Autodesk Fusion 360 part; units mm, degrees
note: some values were not read from the file. Set by a fixed rule: which sketch regions a step uses.
(part 2 of 2)
  circle A929 centre (73.5725, -9.1918) radius 2.5
  circle A930 centre (73.6938, -15.3062) radius 2.5
  circle A931 centre (80.5725, -9.1918) radius 2.5
  point P0 (-62.9957, -145.0372)
  point P1 (82.0043, -145.0372)
  point P2 (-62.9957, -0.0372)
  dimension "d18" = 145
  dimension "d19" = 145
  dimension "d20" = 5
  dimension "d22" = 10
  dimension "d23" = 10
  dimension "d24" = 10
  dimension "d25" = 10
  dimension "d26" = 5
  dimension "d29" = 5
  dimension "d30" = 5
  dimension "d33" = 7
  dimension "d34" = 6
  constraint horizontal L0
  constraint vertical L1
  constraint horizontal L2
  constraint vertical L3
  constraint coincident P0 L0
  constraint coincident P0 L3
  constraint tangent L0 A0
  constraint tangent L3 A0
  constraint coincident P1 L0
  constraint coincident P1 L1
  constraint tangent L0 A1
  constraint tangent L1 A1
  constraint equal A0 A1
  constraint tangent L1 A2
  constraint tangent L2 A2
  constraint equal A0 A2
  constraint coincident P2 L2
  constraint coincident P2 L3
  constraint tangent L2 A3
  constraint tangent L3 A3
  constraint equal A0 A3
  constraint tangent L4 A4
  constraint tangent L7 A4
  constraint tangent L4 A5
  constraint tangent L5 A5
  constraint equal A4 A5
  constraint tangent L5 A6
  constraint tangent L6 A6
  constraint equal A4 A6
  constraint tangent L6 A7
  constraint tangent L7 A7
  constraint equal A4 A7
  measures "d18" distance of P0 P1
  measures "d19" distance of P0 P2
  measures "d20" radius of A0
  measures "d22" distance of L0 L4
  measures "d23" distance of L1 L5
  measures "d24" distance of L2 L6
  measures "d25" distance of L3 L7
  measures "d26" radius of A4
  measures "d29" diameter of A8
  measures "d30" diameter of A9
extrude "Extrude2" add sketch "Sketch2" along normal blind 100 contours L0 L1 L2 L3 A0 A1 A2 A3 A51 A93 A135 A177 A219 A261 A303 A345 A387 A429 A469 A511 A553 A595 A637 A679 A721 A763 A805 A847 A889 A931 | L1 A51 | L1 A93 | L1 A931 | L1 A135 | L1 A889 | L1 A177 | L1 A847 | L1 A219 | L1 A805 | L1 A261 | L1 A763 | L1 A303 | L1 A721 | L1 A345 | L1 A679 | L1 A387 | L1 A637 | L1 A429 | L1 A595 | L1 A469 | L1 A553 | L1 A511 | L4 A15 A58 | A4 A13 A56 | L4 A15 A58 | L4 A15 A58 | A4 A13 A56 | A4 A13 A56 | L4 A17 A60 | A4 A55 A98 | L4 A17 A60 | L4 A17 A60 | L7 A4 A55 A98 | L7 A55 A98 | L4 A19 A62 | L7 A97 A140 | L4 A19 A62 | L4 A19 A62 | L7 A97 A140 | L7 A97 A140 | L4 A21 A64 | L7 A139 A182 | L4 A21 A64 | L4 A21 A64 | L7 A139 A182 | L7 A139 A182 | L4 A23 A66 | L7 A181 A224 | L4 A23 A66 | L4 A23 A66 | L7 A181 A224 | L7 A181 A224 | L4 A25 A68 | L7 A223 A266 | L4 A25 A68 | L4 A25 A68 | L7 A223 A266 | L7 A223 A266 | L4 A27 A70 | L7 A265 A308 | L4 A27 A70 | L4 A27 A70 | L7 A265 A308 | L7 A265 A308 | L4 A29 A72 | L7 A307 A350 | L4 A29 A72 | L4 A29 A72 | L7 A307 A350 | L7 A307 A350 | L4 A31 A74 | L7 A349 A392 | L4 A31 A74 | L4 A31 A74 | L7 A349 A392 | L7 A349 A392 | L4 A33 A76 | L7 A391 A434 | L4 A33 A76 | L4 A33 A76 | L7 A391 A434 | L7 A391 A434 | L4 A35 A78 | L7 A433 A474 | L4 A35 A78 | L4 A35 A78 | L7 A433 A474 | L7 A433 A474 | L4 A37 A80 | L7 A473 A516 | L4 A37 A80 | L4 A37 A80 | L7 A473 A516 | L7 A473 A516 | L4 A39 A82 | L7 A515 A558 | L4 A39 A82 | L4 A39 A82 | L7 A515 A558 | L7 A515 A558 | L4 A41 A84 | L7 A557 A600 | L4 A41 A84 | L4 A41 A84 | L7 A557 A600 | L7 A557 A600 | L4 A43 A86 | L7 A599 A642 | L4 A43 A86 | L4 A43 A86 | L7 A599 A642 | L7 A599 A642 | L4 A45 A88 | L7 A641 A684 | L4 A45 A88 | L4 A45 A88 | L7 A641 A684 | L7 A641 A684 | L4 A47 A90 | L7 A683 A726 | L4 A5 A47 A90 | A5 A47 A90 | L7 A683 A726 | L7 A683 A726 | L5 A5 A91 A134 | L7 A725 A768 | L5 A91 A134 | A91 A134 | L7 A725 A768 | L7 A725 A768 | L5 A133 A176 | L5 A133 A176 | L7 A767 A810 | L5 A133 A176 | L7 A767 A810 | L7 A767 A810 | L5 A175 A218 | L5 A175 A218 | L7 A809 A852 | L5 A175 A218 | L7 A809 A852 | L7 A809 A852 | L5 A217 A260 | L5 A217 A260 | L7 A851 A894 | L5 A217 A260 | L7 A7 A851 A894 | A7 A851 A894 | L5 A259 A302 | L5 A259 A302 | A7 A893 | L5 A259 A302 | L5 A301 A344 | L5 A301 A344 | L6 A895 | L5 A301 A344 | L5 A343 A386 | L6 A897 | L5 A343 A386 | L5 A343 A386 | L6 A899 | L5 A385 A428 | L5 A385 A428 | L6 A901 | L5 A385 A428 | L5 A427 A468 | L6 A903 | L5 A427 A468 | L5 A427 A468 | L6 A905 | L5 A467 A510 | L5 A467 A510 | L6 A907 | L5 A467 A510 | L5 A509 A552 | L6 A909 | L5 A509 A552 | L5 A509 A552 | L6 A911 | L5 A551 A594 | L5 A551 A594 | L6 A913 | L5 A551 A594 | L5 A593 A636 | L6 A915 | L5 A593 A636 | L5 A593 A636 | L6 A917 | L5 A635 A678 | L5 A635 A678 | L6 A919 | L5 A635 A678 | L5 A677 A720 | L6 A921 | L5 A677 A720 | L5 A677 A720 | L6 A923 | L5 A719 A762 | L5 A719 A762 | L6 A925 | L5 A719 A762 | L5 A761 A804 | L6 A6 A927 | L5 A761 A804 | L5 A761 A804 | A6 A887 A930 | L5 A803 A846 | L5 A6 A887 A930 | L5 A887 A930 | L5 A803 A846 | L5 A803 A846 | L5 A845 A888 | L5 A845 A888 | L5 A845 A888 | A11 A54 | A11 A54 | A11 A54 | A12 | A14 | A16 | A18 | A20 | A22 | A24 | A26 | A28 | A30 | A32 | A34 | A36 | A38 | A40 | A42 | A44 | A46 | A48 | A49 A92 | A49 A92 | A49 A92 | A50 | A53 A96 | A53 A96 | A53 A96 | A95 A138 | A95 A138 | A95 A138 | A137 A180 | A137 A180 | A137 A180 | A179 A222 | A179 A222 | A179 A222 | A221 A264 | A221 A264 | A221 A264 | A263 A306 | A263 A306 | A263 A306 | A305 A348 | A305 A348 | A305 A348 | A347 A390 | A347 A390 | A347 A390 | A389 A432 | A389 A432 | A389 A432 | A431 A472 | A431 A472 | A431 A472 | A471 A514 | A471 A514 | A471 A514 | A513 A556 | A513 A556 | A513 A556 | A555 A598 | A555 A598 | A555 A598 | A597 A640 | A597 A640 | A597 A640 | A639 A682 | A639 A682 | A639 A682 | A681 A724 | A681 A724 | A681 A724 | A723 A766 | A723 A766 | A723 A766 | A765 A808 | A765 A808 | A765 A808 | A807 A850 | A807 A850 | A807 A850 | A849 A892 | A849 A892 | A849 A892 | A891 | A929 picked at (80.7025, -135.0711) picked at (80.7025, -129.0711) picked at (80.7025, -9.0711) picked at (80.7025, -123.3125) picked at (80.7025, -15.3125) picked at (80.7025, -117.3125) picked at (80.7025, -21.3125) picked at (80.7025, -111.3125) picked at (80.7025, -27.3125) picked at (80.7025, -105.3125) picked at (80.7025, -33.3125) picked at (80.7025, -99.3125) picked at (80.7025, -39.3125) picked at (80.7025, -93.3125) picked at (80.7717, -45.5438) picked at (80.7025, -87.3125) picked at (80.7717, -51.5438) picked at (80.7025, -81.3125) picked at (80.7025, -57.3125) picked at (80.7025, -75.3125) picked at (80.7025, -63.3125) picked at (80.7025, -69.3125) picked at (-47.8787, -135.1454) picked at (-50.3662, -136.693) picked at (-44.5574, -135.2593) picked at (-43.3662, -136.693) picked at (-53.1044, -135.9845) picked at (-54.0864, -133.4039) picked at (-40.8787, -135.1454) picked at (-52.9107, -131.6684) picked at (-37.5574, -135.2593) picked at (-36.3662, -136.693) picked at (-53.4273, -130.4717) picked at (-54.1416, -127.5346) picked at (-33.8787, -135.1454) picked at (-53.0957, -125.6459) picked at (-30.5574, -135.2593) picked at (-29.3662, -136.693) picked at (-53.1114, -122.5202) picked at (-54.1416, -121.5346) picked at (-26.8787, -135.1454) picked at (-53.0957, -119.6459) picked at (-23.5574, -135.2593) picked at (-22.3662, -136.693) picked at (-53.1114, -116.5202) picked at (-54.1416, -115.5346) picked at (-19.8787, -135.1454) picked at (-53.0957, -113.6459) picked at (-16.5574, -135.2593) picked at (-15.3662, -136.693) picked at (-53.1114, -110.5202) picked at (-54.1416, -109.5346) picked at (-12.8787, -135.1454) picked at (-53.0957, -107.6459) picked at (-9.5574, -135.2593) picked at (-8.3662, -136.693) picked at (-53.1114, -104.5202) picked at (-54.1416, -103.5346) picked at (-5.8787, -135.1454) picked at (-53.0957, -101.6459) picked at (-2.5574, -135.2593) picked at (-1.3662, -136.693) picked at (-53.1114, -98.5202) picked at (-54.1416, -97.5346) picked at (1.1213, -135.1454) picked at (-53.0957, -95.6459) picked at (4.4426, -135.2593) picked at (5.6338, -136.693) picked at (-53.1114, -92.5202) picked at (-54.1416, -91.5346) picked at (8.1213, -135.1454) picked at (-53.0957, -89.6459) picked at (11.4426, -135.2593) picked at (12.6338, -136.693) picked at (-53.1114, -86.5202) picked at (-54.1416, -85.5346) picked at (15.1213, -135.1454) picked at (-53.0957, -83.6459) picked at (18.4426, -135.2593) picked at (19.6338, -136.693) picked at (-53.1114, -80.5202) picked at (-54.1416, -79.5346) picked at (22.1213, -135.1454) picked at (-53.0957, -77.6459) picked at (25.4426, -135.2593) picked at (26.6338, -136.693) picked at (-53.1114, -74.5202) picked at (-54.1416, -73.5346) picked at (29.1213, -135.1454) picked at (-53.0957, -71.6459) picked at (32.4426, -135.2593) picked at (33.6338, -136.693) picked at (-53.1114, -68.5202) picked at (-54.1416, -67.5346) picked at (36.1213, -135.1454) picked at (-53.0957, -65.6459) picked at (39.4426, -135.2593) picked at (40.6338, -136.693) picked at (-53.1114, -62.5202) picked at (-54.1416, -61.5346) picked at (43.1213, -135.1454) picked at (-53.0957, -59.6459) picked at (46.4426, -135.2593) picked at (47.6338, -136.693) picked at (-53.1114, -56.5202) picked at (-54.1416, -55.5346) picked at (50.1213, -135.1454) picked at (-53.0957, -53.6459) picked at (53.4426, -135.2593) picked at (54.6338, -136.693) picked at (-53.1114, -50.5202) picked at (-54.1416, -49.5346) picked at (57.1213, -135.1454) picked at (-53.0957, -47.6459) picked at (60.4426, -135.2593) picked at (61.6338, -136.693) picked at (-53.1114, -44.5202) picked at (-54.1416, -43.5346) picked at (64.1213, -135.1454) picked at (-53.0957, -41.6459) picked at (67.6322, -135.7046) picked at (68.6338, -136.693) picked at (-53.1114, -38.5202) picked at (-54.1416, -37.5346) picked at (-53.0957, -35.6459) picked at (72.1, -127.315) picked at (-53.1114, -32.5202) picked at (-54.1416, -31.5346) picked at (75.2803, -125.0858) picked at (74.178, -123.836) picked at (-53.0957, -29.6459) picked at (72.1, -121.315) picked at (-53.1114, -26.5202) picked at (-54.1416, -25.5346) picked at (75.2803, -119.0858) picked at (74.178, -117.836) picked at (-53.0957, -23.6459) picked at (72.1, -115.315) picked at (-53.1114, -20.5202) picked at (-54.1416, -19.5346) picked at (75.2803, -113.0858) picked at (74.178, -111.836) picked at (-53.0957, -17.6459) picked at (72.1, -109.315) picked at (-53.5343, -14.6405) picked at (-54.2241, -13.6237) picked at (75.2803, -107.0858) picked at (74.178, -105.836) picked at (-51.9972, -9.7788) picked at (72.1, -103.315) picked at (75.2803, -101.0858) picked at (74.178, -99.836) picked at (-44.6616, -9.4001) picked at (72.1, -97.315) picked at (75.2803, -95.0858) picked at (-37.6616, -9.4001) picked at (74.178, -93.836) picked at (72.1, -91.315) picked at (-30.7199, -9.1671) picked at (75.2803, -89.0858) picked at (74.178, -87.836) picked at (-23.6355, -9.5182) picked at (72.1, -85.315) picked at (75.2803, -83.0858) picked at (-16.7534, -8.2075) picked at (74.178, -81.836) picked at (72.1, -79.315) picked at (-10.2431, -8.8343) picked at (75.2803, -77.0858) picked at (74.178, -75.836) picked at (-3.4827, -8.8058) picked at (72.1, -73.315) picked at (75.2803, -71.0858) picked at (4.163, -9.0854) picked at (74.178, -69.836) picked at (72.1, -67.315) picked at (10.6228, -8.6914) picked at (75.2803, -65.0858) picked at (74.178, -63.836) picked at (16.6268, -7.9596) picked at (72.1, -61.315) picked at (75.2803, -59.0858) picked at (25.2637, -9.0896) picked at (74.178, -57.836) picked at (72.1, -55.315) picked at (31.9561, -7.9363) picked at (75.2803, -53.0858) picked at (74.178, -51.836) picked at (37.8068, -8.9263) picked at (72.1, -49.315) picked at (75.2803, -47.0858) picked at (45.9286, -7.8781) picked at (74.178, -45.836) picked at (72.1, -43.315) picked at (52.9286, -7.8781) picked at (75.2803, -41.0858) picked at (74.178, -39.836) picked at (58.8068, -8.9263) picked at (72.1, -37.315) picked at (75.2803, -35.0858) picked at (67.7582, -9.3101) picked at (74.178, -33.836) picked at (72.1, -31.315) picked at (72.1469, -13.2786) picked at (75.2803, -29.0858) picked at (74.2093, -13.9759) picked at (75.2803, -17.0858) picked at (74.178, -27.836) picked at (72.1, -25.315) picked at (72.1, -19.315) picked at (75.2803, -23.0858) picked at (74.178, -21.836) makes body 1
extrude "Extrude3" add sketch "Sketch2" along normal blind 2 contours L4 L5 L6 L7 A4 A5 A6 A7 A13 A15 A17 A19 A21 A23 A25 A27 A29 A31 A33 A35 A37 A39 A41 A43 A45 A47 A55 A56 A58 A60 A62 A64 A66 A68 A70 A72 A74 A76 A78 A80 A82 A84 A86 A88 A90 A91 A97 A98 A133 A139 A140 A175 A176 A181 A182 A217 A218 A223 A224 A259 A260 A265 A266 A301 A302 A307 A308 A343 A344 A349 A350 A385 A386 A391 A392 A427 A428 A433 A434 A467 A468 A473 A474 A509 A510 A515 A516 A551 A552 A557 A558 A593 A594 A599 A600 A635 A636 A641 A642 A677 A678 A683 A684 A719 A720 A725 A726 A761 A762 A767 A768 A803 A804 A809 A810 A845 A846 A851 A852 A887 A888 A893 A894 A895 A897 A899 A901 A903 A905 A907 A909 A911 A913 A915 A917 A919 A921 A923 A925 A927 A930 bodies 1
sketch "Sketch6" plane through (0, 100, 0) normal (0, 1, 0) x (-1, 0, 0)
  arc A0 (47.9957, 10.0372) -> (52.9957, 15.0372) centre (47.9957, 15.0372) ccw
  line L0 (47.9957, 10.0372) -> (-67.0043, 10.0372)
  arc A1 (-72.0043, 15.0372) -> (-67.0043, 10.0372) centre (-67.0043, 15.0372) ccw
  line L1 (-72.0043, 15.0372) -> (-72.0043, 130.0372)
  arc A2 (-67.0043, 135.0372) -> (-72.0043, 130.0372) centre (-67.0043, 130.0372) ccw
  line L2 (-67.0043, 135.0372) -> (47.9957, 135.0372)
  arc A3 (52.9957, 130.0372) -> (47.9957, 135.0372) centre (47.9957, 130.0372) ccw
  line L3 (52.9957, 130.0372) -> (52.9957, 15.0372)
  arc A4 (57.9957, 0.0372) -> (62.9957, 5.0372) centre (57.9957, 5.0372) ccw
  line L4 (62.9957, 5.0372) -> (62.9957, 140.0372)
  arc A5 (62.9957, 140.0372) -> (57.9957, 145.0372) centre (57.9957, 140.0372) ccw
  line L5 (57.9957, 145.0372) -> (-77.0043, 145.0372)
  arc A6 (-77.0043, 145.0372) -> (-82.0043, 140.0372) centre (-77.0043, 140.0372) ccw
  line L6 (-82.0043, 140.0372) -> (-82.0043, 5.0372)
  arc A7 (-82.0043, 5.0372) -> (-77.0043, 0.0372) centre (-77.0043, 5.0372) ccw
  line L7 (-77.0043, 0.0372) -> (57.9957, 0.0372)
  line L8 (-77.0377, 145.0391) -> (57.9623, 145.0391)
  line L9 (62.9623, 140.0391) -> (62.9623, 5.0391)
  line L10 (57.9623, 0.0391) -> (-77.0377, 0.0391)
  line L11 (-82.0377, 5.0391) -> (-82.0377, 140.0391)
  arc A8 (-77.0377, 145.0391) -> (-82.0377, 140.0391) centre (-77.0377, 140.0391) ccw
  arc A9 (62.9623, 140.0391) -> (57.9623, 145.0391) centre (57.9623, 140.0391) ccw
  arc A10 (57.9623, 0.0391) -> (62.9623, 5.0391) centre (57.9623, 5.0391) ccw
  arc A11 (-82.0377, 5.0391) -> (-77.0377, 0.0391) centre (-77.0377, 5.0391) ccw
  point P0 (-82.0377, 145.0391)
  point P1 (62.9623, 145.0391)
  point P2 (-82.0377, 0.0391)
  dimension "d39" = 145
  dimension "d40" = 145
  dimension "d41" = 5
  constraint horizontal L8
  constraint vertical L9
  constraint horizontal L10
  constraint vertical L11
  constraint coincident P0 L8
  constraint coincident P0 L11
  constraint tangent L8 A8
  constraint tangent L11 A8
  constraint coincident P1 L8
  constraint coincident P1 L9
  constraint tangent L8 A9
  constraint tangent L9 A9
  constraint equal A8 A9
  constraint tangent L9 A10
  constraint tangent L10 A10
  constraint equal A8 A10
  constraint coincident P2 L10
  constraint coincident P2 L11
  constraint tangent L10 A11
  constraint tangent L11 A11
  constraint equal A8 A11
  measures "d39" distance of P0 P1
  measures "d40" distance of P0 P2
  measures "d41" radius of A8
move_body "Move1" bodies 1 to x (1, 0, 0) y (0, 1, 0) z (0, 0, 1) at (0, -40, 0)
extrude "Extrude4" add sketch "Sketch6" along normal blind 2.5 separate body contours A0 L0 A1 L1 A2 L2 A3 L3 | L5 A6 L6 A7 L7 L8 L9 L10 A9 A10 makes body 2
move_body "Move2" bodies 2 to x (1, 0, 0) y (0, 1, 0) z (0, 0, 1) at (250, -110, 0)
sketch "Sketch7" plane through (0, 0, 10.0372) normal (0, 0, 1) x (-1, 0, 0)
  line L0 (47.7802, 38) -> (47.7802, 40)
  line L1 (47.7802, 40) -> (43.0748, 40)
  line L2 (43.0748, 40) -> (43.0748, 38)
  line L3 (43.0748, 38) -> (40.7802, 38)
  line L4 (40.7802, 38) -> (40.7802, 40)
  line L5 (40.7802, 40) -> (36.0748, 40)
  line L6 (36.0748, 40) -> (36.0748, 38)
  line L7 (36.0748, 38) -> (33.7802, 38)
  line L8 (33.7802, 38) -> (33.7802, 40)
  line L9 (33.7802, 40) -> (29.0748, 40)
  line L10 (29.0748, 40) -> (29.0748, 38)
  line L11 (29.0748, 38) -> (26.7802, 38)
  line L12 (26.7802, 38) -> (26.7802, 40)
  line L13 (26.7802, 40) -> (22.0748, 40)
  line L14 (22.0748, 40) -> (22.0748, 38)
  line L15 (22.0748, 38) -> (19.7802, 38)
  line L16 (19.7802, 38) -> (19.7802, 40)
  line L17 (19.7802, 40) -> (15.0748, 40)
  line L18 (15.0748, 40) -> (15.0748, 38)
  line L19 (15.0748, 38) -> (12.7802, 38)
  line L20 (12.7802, 38) -> (12.7802, 40)
  line L21 (12.7802, 40) -> (8.0748, 40)
  line L22 (8.0748, 40) -> (8.0748, 38)
  line L23 (8.0748, 38) -> (5.7802, 38)
  line L24 (5.7802, 38) -> (5.7802, 40)
  line L25 (5.7802, 40) -> (1.0748, 40)
  line L26 (1.0748, 40) -> (1.0748, 38)
  line L27 (1.0748, 38) -> (-1.2198, 38)
  line L28 (-1.2198, 38) -> (-1.2198, 40)
  line L29 (-1.2198, 40) -> (-5.9252, 40)
  line L30 (-5.9252, 40) -> (-5.9252, 38)
  line L31 (-5.9252, 38) -> (-8.2198, 38)
  line L32 (-8.2198, 38) -> (-8.2198, 40)
  line L33 (-8.2198, 40) -> (-12.9252, 40)
  line L34 (-12.9252, 40) -> (-12.9252, 38)
  line L35 (-12.9252, 38) -> (-15.2198, 38)
  line L36 (-15.2198, 38) -> (-15.2198, 40)
  line L37 (-15.2198, 40) -> (-19.9252, 40)
  line L38 (-19.9252, 40) -> (-19.9252, 38)
  line L39 (-19.9252, 38) -> (-22.2198, 38)
  line L40 (-22.2198, 38) -> (-22.2198, 40)
  line L41 (-22.2198, 40) -> (-26.9252, 40)
  line L42 (-26.9252, 40) -> (-26.9252, 38)
  line L43 (-26.9252, 38) -> (-29.2198, 38)
  line L44 (-29.2198, 38) -> (-29.2198, 40)
  line L45 (-29.2198, 40) -> (-33.9252, 40)
  line L46 (-33.9252, 40) -> (-33.9252, 38)
  line L47 (-33.9252, 38) -> (-36.2198, 38)
  line L48 (-36.2198, 38) -> (-36.2198, 40)
  line L49 (-36.2198, 40) -> (-40.9252, 40)
  line L50 (-40.9252, 40) -> (-40.9252, 38)
  line L51 (-40.9252, 38) -> (-43.2198, 38)
  line L52 (-43.2198, 38) -> (-43.2198, 40)
  line L53 (-43.2198, 40) -> (-47.9252, 40)
  line L54 (-47.9252, 40) -> (-47.9252, 38)
  line L55 (-47.9252, 38) -> (-50.2198, 38)
  line L56 (-50.2198, 38) -> (-50.2198, 40)
  line L57 (-50.2198, 40) -> (-54.9252, 40)
  line L58 (-54.9252, 40) -> (-54.9252, 38)
  line L59 (-54.9252, 38) -> (-57.2198, 38)
  line L60 (-57.2198, 38) -> (-57.2198, 40)
  line L61 (-57.2198, 40) -> (-61.9252, 40)
  line L62 (-61.9252, 40) -> (-61.9252, 38)
  line L63 (-61.9252, 38) -> (-64.2198, 38)
  line L64 (-64.2198, 38) -> (-64.2198, 40)
  line L65 (-64.2198, 40) -> (-67.0043, 40)
  line L66 (-67.0043, 40) -> (-67.0043, -60)
  line L67 (-67.0043, -60) -> (47.9957, -60)
  line L68 (47.9957, -60) -> (47.9957, 38)
  line L69 (47.9957, 38) -> (47.7802, 38)
  line L70 (-49.5, 15) -> (30.5, 15)
  line L71 (30.5, 15) -> (30.5, -35)
  line L72 (30.5, -35) -> (-49.5, -35)
  line L73 (-49.5, -35) -> (-49.5, 15)
  dimension "d44" = 80
  dimension "d45" = 50
  constraint horizontal L70
  constraint vertical L71
  constraint horizontal L72
  constraint vertical L73
  measures "d44" distance of L70.start L70.end
  measures "d45" distance of L70.start L72.end
extrude "Extrude5" add sketch "Sketch7" along normal blind 20 contours L70 L71 L72 L73 bodies 1
sketch "Sketch9" plane through (0, 60, 0) normal (0, 1, 0) x (-1, 0, 0)
  arc A0 (47.9957, 10.0372) -> (52.9957, 15.0372) centre (47.9957, 15.0372) ccw
  line L0 (47.9957, 10.0372) -> (-67.0043, 10.0372)
  arc A1 (-72.0043, 15.0372) -> (-67.0043, 10.0372) centre (-67.0043, 15.0372) ccw
  line L1 (-72.0043, 15.0372) -> (-72.0043, 130.0372)
  arc A2 (-67.0043, 135.0372) -> (-72.0043, 130.0372) centre (-67.0043, 130.0372) ccw
  line L2 (-67.0043, 135.0372) -> (47.9957, 135.0372)
  arc A3 (52.9957, 130.0372) -> (47.9957, 135.0372) centre (47.9957, 130.0372) ccw
  line L3 (52.9957, 130.0372) -> (52.9957, 15.0372)
  arc A4 (57.9957, 0.0372) -> (62.9957, 5.0372) centre (57.9957, 5.0372) ccw
  line L4 (62.9957, 5.0372) -> (62.9957, 140.0372)
  arc A5 (62.9957, 140.0372) -> (57.9957, 145.0372) centre (57.9957, 140.0372) ccw
  line L5 (57.9957, 145.0372) -> (-77.0043, 145.0372)
  arc A6 (-77.0043, 145.0372) -> (-82.0043, 140.0372) centre (-77.0043, 140.0372) ccw
  line L6 (-82.0043, 140.0372) -> (-82.0043, 5.0372)
  arc A7 (-82.0043, 5.0372) -> (-77.0043, 0.0372) centre (-77.0043, 5.0372) ccw
  line L7 (-77.0043, 0.0372) -> (57.9957, 0.0372)
sketch "Sketch10" plane through (0, -7.5, 0) normal (0, 1, 0) x (-1, 0, 0)
sketch "Sketch11" plane through (0, 0, 0) normal (0, 1, 0) x (1, 0, 0)
  line L0 (-119.9551, 0) -> (-254.9551, 0)
  line L1 (-259.9551, -5) -> (-259.9551, -140)
  line L2 (-254.9551, -145) -> (-119.9551, -145)
  line L3 (-114.9551, -140) -> (-114.9551, -5)
  line L4 (-249.9551, -15) -> (-249.9551, -130)
  line L5 (-244.9551, -135) -> (-129.9551, -135)
  line L6 (-124.9551, -130) -> (-124.9551, -15)
  line L7 (-129.9551, -10) -> (-244.9551, -10)
  arc A0 (-129.9551, -135) -> (-124.9551, -130) centre (-129.9551, -130) ccw
  arc A1 (-249.9551, -130) -> (-244.9551, -135) centre (-244.9551, -130) ccw
  arc A2 (-244.9551, -10) -> (-249.9551, -15) centre (-244.9551, -15) ccw
  arc A3 (-124.9551, -15) -> (-129.9551, -10) centre (-129.9551, -15) ccw
  arc A4 (-114.9551, -5) -> (-119.9551, 0) centre (-119.9551, -5) ccw
  arc A5 (-254.9551, 0) -> (-259.9551, -5) centre (-254.9551, -5) ccw
  arc A6 (-259.9551, -140) -> (-254.9551, -145) centre (-254.9551, -140) ccw
  arc A7 (-119.9551, -145) -> (-114.9551, -140) centre (-119.9551, -140) ccw
  point P0 (-114.9551, 0)
  point P1 (-259.9551, 0)
  point P2 (-114.9551, -145)
  dimension "d48" = 145
  dimension "d49" = 145
  dimension "d51" = 10
  dimension "d52" = 10
  dimension "d53" = 10
  dimension "d54" = 10
  dimension "d55" = 5
  constraint horizontal L0
  constraint vertical L1
  constraint horizontal L2
  constraint vertical L3
  constraint tangent L5 A0
  constraint tangent L6 A0
  constraint tangent L4 A1
  constraint tangent L5 A1
  constraint equal A0 A1
  constraint tangent L4 A2
  constraint tangent L7 A2
  constraint equal A0 A2
  constraint tangent L6 A3
  constraint tangent L7 A3
  constraint equal A0 A3
  constraint coincident P0 L0
  constraint coincident P0 L3
  constraint tangent L0 A4
  constraint tangent L3 A4
  constraint equal A0 A4
  constraint coincident P1 L0
  constraint coincident P1 L1
  constraint tangent L0 A5
  constraint tangent L1 A5
  constraint equal A0 A5
  constraint tangent L1 A6
  constraint tangent L2 A6
  constraint equal A0 A6
  constraint coincident P2 L2
  constraint coincident P2 L3
  constraint tangent L2 A7
  constraint tangent L3 A7
  constraint equal A0 A7
  measures "d48" distance of P0 P1
  measures "d49" distance of P0 P2
  measures "d51" distance of L1 L4
  measures "d52" distance of L2 L5
  measures "d53" distance of L3 L6
  measures "d54" distance of L0 L7
  measures "d55" radius of A0
extrude "Extrude6" cut sketch "Sketch9" against normal blind 20 bodies 1
extrude "Extrude7" add sketch "Sketch11" along normal blind 70 separate body makes body 3
move_body "Move3" bodies 3 to x (1, 0, 0) y (0, 1, 0) z (0, 0, 1) at (196.9061, 59.5351, 0)
move_body "Move4" bodies 3 to x (1, 0, 0) y (0, 1, 0) z (0, 0, 1) at (0, 30, 0)
move_body "Move5" bodies 1 to x (-1, 0, 0) y (0, -1, 0) z (0, 0, 1) at (19.0086, 0, 0)
move_body "Move6" bodies 3 to x (1, 0, 0) y (0, 1, 0) z (0, 0, 1) at (0, -250, 0)
move_body "Move7" bodies 2 to x (1, 0, 0) y (0, 1, 0) z (0, 0, 1) at (-250, -205, 0)
move_body "Move8" bodies 2 to x (1, 0, 0) y (0, 1, 0) z (0, 0, 1) at (0, -110, 0)
move_body "Move9" bodies 3 to x (1, 0, 0) y (0, 1, 0) z (0, 0, 1) at (0, -30, 0)
move_body "Move10" bodies 2 to x (1, 0, 0) y (0, 1, 0) z (0, 0, 1) at (0, 40, 0)
sketch "Sketch12" plane through (0, -285, 0) normal (0, -1, 0) x (1, 0, 0)
  arc A0 (-58.2645, 145.0299) -> (-62.9623, 140.0391) centre (-57.9623, 140.0391) ccw
  line L0 (-62.9623, 140.0391) -> (-62.9623, 5.0391)
  arc A1 (-62.9623, 5.0391) -> (-57.9623, 0.0391) centre (-57.9623, 5.0391) ccw
  line L1 (-57.9623, 0.0391) -> (77.0377, 0.0391)
  arc A2 (77.0377, 0.0391) -> (77.3066, 0.0463) centre (77.0377, 5.0391) ccw
  arc A3 (77.3066, 0.0463) -> (82.0043, 5.0372) centre (77.0043, 5.0372) ccw
  line L2 (82.0043, 5.0372) -> (82.0043, 140.0372)
  arc A4 (82.0043, 140.0372) -> (77.0043, 145.0372) centre (77.0043, 140.0372) ccw
  line L3 (77.0043, 145.0372) -> (-57.9957, 145.0372)
  arc A5 (-57.9957, 145.0372) -> (-58.2645, 145.0299) centre (-57.9957, 140.0372) ccw
  line L4 (13.1379, 11.0093) -> (5.8379, 11.0093)
  line L5 (4.8379, 12.0093) -> (4.8379, 13.6093)
  line L6 (5.8379, 14.6093) -> (13.1379, 14.6093)
  line L7 (14.1379, 13.6093) -> (14.1379, 12.0093)
  arc A6 (5.8379, 14.6093) -> (4.8379, 13.6093) centre (5.8379, 13.6093) ccw
  arc A7 (14.1379, 13.6093) -> (13.1379, 14.6093) centre (13.1379, 13.6093) ccw
  arc A8 (13.1379, 11.0093) -> (14.1379, 12.0093) centre (13.1379, 12.0093) ccw
  arc A9 (4.8379, 12.0093) -> (5.8379, 11.0093) centre (5.8379, 12.0093) ccw
  point P0 (14.1379, 11.0093)
  point P1 (4.8379, 11.0093)
  point P2 (14.1379, 14.6093)
  dimension "d60" = 9.3
  dimension "d61" = 3.6
  dimension "d62" = 1
  constraint horizontal L4
  constraint vertical L5
  constraint horizontal L6
  constraint vertical L7
  constraint tangent L5 A6
  constraint tangent L6 A6
  constraint coincident P2 L6
  constraint coincident P2 L7
  constraint tangent L6 A7
  constraint tangent L7 A7
  constraint equal A6 A7
  constraint coincident P0 L4
  constraint coincident P0 L7
  constraint tangent L4 A8
  constraint tangent L7 A8
  constraint equal A6 A8
  constraint coincident P1 L4
  constraint coincident P1 L5
  constraint tangent L4 A9
  constraint tangent L5 A9
  constraint equal A6 A9
  measures "d60" distance of P0 P1
  measures "d61" distance of P0 P2
  measures "d62" radius of A6
extrude "Extrude8" cut sketch "Sketch12" against normal blind 2.5 contours L4 L5 L6 L7 A6 A7 A8 A9 bodies 2
sketch "Sketch14" plane through (0, -285, 0) normal (0, -1, 0) x (1, 0, 0)
  line L0 (4.8379, 12.0093) -> (4.8379, 13.6093)
  arc A0 (5.8379, 14.6093) -> (4.8379, 13.6093) centre (5.8379, 13.6093) ccw
  line L1 (5.8379, 14.6093) -> (13.1379, 14.6093)
  arc A1 (14.1379, 13.6093) -> (13.1379, 14.6093) centre (13.1379, 13.6093) ccw
  line L2 (14.1379, 13.6093) -> (14.1379, 12.0093)
  arc A2 (13.1379, 11.0093) -> (14.1379, 12.0093) centre (13.1379, 12.0093) ccw
  line L3 (13.1379, 11.0093) -> (5.8379, 11.0093)
  arc A3 (4.8379, 12.0093) -> (5.8379, 11.0093) centre (5.8379, 12.0093) ccw
  arc A4 (-58.2645, 145.0299) -> (-62.9623, 140.0391) centre (-57.9623, 140.0391) ccw
  line L4 (-62.9623, 140.0391) -> (-62.9623, 5.0391)
  arc A5 (-62.9623, 5.0391) -> (-57.9623, 0.0391) centre (-57.9623, 5.0391) ccw
  line L5 (-57.9623, 0.0391) -> (77.0377, 0.0391)
  arc A6 (77.0377, 0.0391) -> (77.3066, 0.0463) centre (77.0377, 5.0391) ccw
  arc A7 (77.3066, 0.0463) -> (82.0043, 5.0372) centre (77.0043, 5.0372) ccw
  line L6 (82.0043, 5.0372) -> (82.0043, 140.0372)
  arc A8 (82.0043, 140.0372) -> (77.0043, 145.0372) centre (77.0043, 140.0372) ccw
  line L7 (77.0043, 145.0372) -> (-57.9957, 145.0372)
  arc A9 (-57.9957, 145.0372) -> (-58.2645, 145.0299) centre (-57.9957, 140.0372) ccw
  line L8 (-47.7061, 133.5938) -> (67.2939, 133.5938)
  line L9 (72.2939, 128.5938) -> (72.2939, 28.1938)
  line L10 (67.2939, 23.1938) -> (-47.7061, 23.1938)
  line L11 (-52.7061, 28.1938) -> (-52.7061, 128.5938)
  arc A10 (-47.7061, 133.5938) -> (-52.7061, 128.5938) centre (-47.7061, 128.5938) ccw
  arc A11 (72.2939, 128.5938) -> (67.2939, 133.5938) centre (67.2939, 128.5938) ccw
  arc A12 (67.2939, 23.1938) -> (72.2939, 28.1938) centre (67.2939, 28.1938) ccw
  arc A13 (-52.7061, 28.1938) -> (-47.7061, 23.1938) centre (-47.7061, 28.1938) ccw
  point P0 (-52.7061, 133.5938)
  point P1 (72.2939, 133.5938)
  point P2 (-52.7061, 23.1938)
  dimension "d67" = 125
  dimension "d68" = 110.4
  dimension "d69" = 5
  constraint horizontal L8
  constraint vertical L9
  constraint horizontal L10
  constraint vertical L11
  constraint coincident P0 L8
  constraint coincident P0 L11
  constraint tangent L8 A10
  constraint tangent L11 A10
  constraint coincident P1 L8
  constraint coincident P1 L9
  constraint tangent L8 A11
  constraint tangent L9 A11
  constraint equal A10 A11
  constraint tangent L9 A12
  constraint tangent L10 A12
  constraint equal A10 A12
  constraint coincident P2 L10
  constraint coincident P2 L11
  constraint tangent L10 A13
  constraint tangent L11 A13
  constraint equal A10 A13
  measures "d67" distance of P0 P1
  measures "d68" distance of P0 P2
  measures "d69" radius of A10
extrude "Extrude9" cut sketch "Sketch14" against normal blind 2.5 contours L8 L9 L10 L11 A10 A11 A12 A13 bodies 2
move_body "Move11" bodies 3 to x (1, 0, 0) y (0, 1, 0) z (0, 0, 1) at (0, 80.5, 0)
move_body "Move12" bodies 2 to x (1, 0, 0) y (0, 1, 0) z (0, 0, 1) at (-0.1, 172.6, 0)
